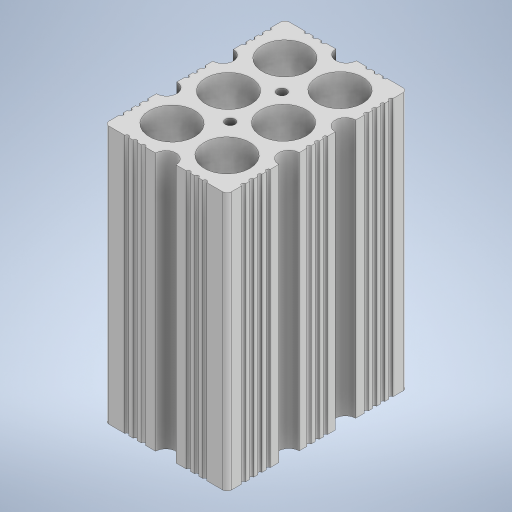
# Autodesk Inventor part: Tijolo 9x19cm
Saved by Autodesk Inventor 2024.4 (Build 284460000, 460)
## iProperties
Created: 2026-08-26
Part Number: Tijolo 9x19cm
Material: Generic
Document SubType Name: Modeling
Designer: MaryPinkAssus
Density: 1 g/cm^3
Appearance: Default
Author: MaryPinkAssus
Autodesk Inventor part; units mm, degrees
ref_plane "YZ Plane" through (0, 0, 0) normal (1, 0, 0) x (0, 1, 0)
ref_plane "XZ Plane" through (0, 0, 0) normal (0, 1, 0) x (-1, 0, 0)
ref_plane "XY Plane" through (0, 0, 0) normal (0, 0, 1) x (1, 0, 0)
sketch "Sketch1" plane through (0, 0, 0) normal (0, 0, 1) x (1, 0, 0)
  line L0 (0, 0) -> (89.5, 0)
  line L1 (89.5, 0) -> (89.5, 188.8)
  line L2 (89.5, 188.8) -> (0, 188.8)
  line L3 (0, 188.8) -> (0, 0)
  dimension "d0" = 89.5
  dimension "d1" = 188.8
  constraints: 8 end point, 2 parallel, 1 horizontal, 1 perpendicular
  measures "d0" distance of L2.end L1.end
  measures "d1" distance of L1.end L0.end
extrude "Corpo" add sketch "Sketch1" along normal blind 131.8
sketch "Furações" plane through (0, 0, 0) normal (0, -1, 0) x (1, 0, 0)
  line L0 (89.5, 131.8) -> (0, 131.8) projected
  line L1 (89.5, 0) -> (0, 0) projected
  line L2 (44.75, 131.8) -> (44.75, 84.8) construction
  line L3 (44.75, 0) -> (44.75, 47) construction
  circle A0 centre (44.75, 84.8) radius 3.5
  circle A1 centre (44.75, 47) radius 3.5
  line L4 (89.5, 123.8) -> (0, 123.8) construction
  line L5 (8, 0) -> (8, 131.8) construction
  line L6 (41.25, 131.8) -> (41.25, 84.8) construction
  circle A2 centre (24.625, 107.175) radius 16.625
  line L7 (0, 0) -> (0, 131.8) construction
  line L8 (0, 65.9) -> (89.5, 65.9) construction
  line L9 (89.5, 0) -> (89.5, 131.8) projected
  line L10 (24.625, 131.8) -> (156.425, 131.8) construction
  circle A3 centre (24.625, 65.9) radius 16.625
  line L11 (0, 8) -> (89.5, 8) construction
  line L12 (41.25, 0) -> (41.25, 47) construction
  circle A4 centre (24.625, 24.625) radius 16.625
  circle A5 centre (64.875, 107.175) radius 16.625
  circle A6 centre (64.875, 65.9) radius 16.625
  circle A7 centre (64.875, 24.625) radius 16.625
  circle A8 centre (44.75, 131.8) radius 7.5
  circle A9 centre (44.75, 0) radius 7.5
  line L13 (24.625, 131.8) -> (24.625, 123.8) construction
  line L14 (24.625, 90.55) -> (24.625, 82.525) construction
  line L15 (24.625, 49.275) -> (24.625, 41.25) construction
  line L16 (24.625, 8) -> (24.625, 0) construction
  line L17 (24.625, 86.5375) -> (0, 86.5375) construction
  line L18 (24.625, 45.2625) -> (0, 45.2625) construction
  circle A10 centre (0, 86.5375) radius 7.5
  circle A11 centre (0, 45.2625) radius 7.5
  circle A12 centre (89.5, 86.5375) radius 7.5
  circle A13 centre (89.5, 45.2625) radius 7.5
  line L19 (0, 123.8) -> (0, 119.8) construction
  circle A14 centre (0, 119.8) radius 1.5
  line L20 (0, 119.8) -> (0, 113.8) construction
  circle A15 centre (0, 113.8) radius 1.5
  line L21 (0, 113.8) -> (0, 107.8) construction
  circle A16 centre (0, 107.8) radius 1.5
  line L22 (0, 107.8) -> (0, 101.8) construction
  circle A17 centre (0, 101.8) radius 1.5
  circle A18 centre (0, 65.9) radius 1.5
  line L23 (0, 65.9) -> (0, 71.9) construction
  line L24 (0, 65.9) -> (0, 59.9) construction
  circle A19 centre (0, 71.9) radius 1.5
  circle A20 centre (0, 59.9) radius 1.5
  line L25 (0, 8) -> (0, 12) construction
  circle A21 centre (0, 12) radius 1.5
  line L26 (0, 12) -> (0, 18) construction
  circle A22 centre (0, 18) radius 1.5
  line L27 (0, 18) -> (0, 24) construction
  circle A23 centre (0, 24) radius 1.5
  line L28 (0, 24) -> (0, 30) construction
  circle A24 centre (0, 30) radius 1.5
  line L29 (37.25, 0) -> (28.25, 0) construction
  circle A25 centre (28.25, 0) radius 1.5
  line L30 (28.25, 0) -> (22.25, 0) construction
  circle A26 centre (22.25, 0) radius 1.5
  line L31 (22.25, 0) -> (16.25, 0) construction
  circle A27 centre (16.25, 0) radius 1.5
  circle A28 centre (28.25, 131.8) radius 1.5
  line L32 (28.25, 131.8) -> (22.25, 131.8) construction
  circle A29 centre (22.25, 131.8) radius 1.5
  line L33 (22.25, 131.8) -> (16.25, 131.8) construction
  circle A30 centre (16.25, 131.8) radius 1.5
  circle A31 centre (89.5, 119.8) radius 1.5
  circle A32 centre (89.5, 113.8) radius 1.5
  circle A33 centre (89.5, 107.8) radius 1.5
  circle A34 centre (89.5, 101.8) radius 1.5
  circle A35 centre (89.5, 65.9) radius 1.5
  circle A36 centre (89.5, 71.9) radius 1.5
  circle A37 centre (89.5, 59.9) radius 1.5
  circle A38 centre (89.5, 12) radius 1.5
  circle A39 centre (89.5, 18) radius 1.5
  circle A40 centre (89.5, 24) radius 1.5
  circle A41 centre (89.5, 30) radius 1.5
  circle A42 centre (61.25, 0) radius 1.5
  circle A43 centre (67.25, 0) radius 1.5
  circle A44 centre (73.25, 0) radius 1.5
  circle A45 centre (73.25, 131.8) radius 1.5
  circle A46 centre (67.25, 131.8) radius 1.5
  circle A47 centre (61.25, 131.8) radius 1.5
  dimension "d4" = 47
  dimension "d5" = 47
  dimension "d6" = 7
  dimension "d7" = 7
  dimension "d8" = 8
  dimension "d9" = 8
  dimension "d10" = 3.5
  dimension "d12" = 33.25
  dimension "d13" = 3.5
  dimension "d14" = 15
  dimension "d15" = 15
  dimension "d16" = 15
  dimension "d17" = 4
  dimension "d18" = 3
  dimension "d19" = 6
  dimension "d20" = 3
  dimension "d21" = 6
  dimension "d22" = 3
  dimension "d23" = 6
  dimension "d24" = 3
  dimension "d25" = 3
  dimension "d26" = 6
  dimension "d27" = 6
  dimension "d28" = 3
  dimension "d29" = 3
  dimension "d30" = 4
  dimension "d31" = 3
  dimension "d32" = 6
  dimension "d33" = 3
  dimension "d34" = 6
  dimension "d35" = 3
  dimension "d36" = 6
  dimension "d37" = 3
  dimension "d38" = 9
  dimension "d39" = 3
  dimension "d40" = 6
  dimension "d41" = 3
  dimension "d42" = 6
  dimension "d43" = 3
  constraints: 60 end point, 47 centre point, 29 symmetric about line, 22 coincident, 6 point on circle, 6 tangent, 4 midpoint, 3 horizontal, 3 parallel, 3 point on line, 2 perpendicular, 1 horizontal alignment, 51 other
  measures "d4" distance of L2.start L2.end
  measures "d5" distance of L3.start L3.end
  measures "d6" diameter of A0
  measures "d7" diameter of A1
  measures "d8" distance between parallel lines of L0 L4
  measures "d9" distance of point (0, 0) L5.start
  measures "d10" distance between parallel lines of L2 L6
  measures "d12" diameter of A3
  measures "d13" distance between parallel lines of L3 L12
  measures "d14" diameter of A8
  measures "d15" diameter of A10
  measures "d16" diameter of A11
  measures "d17" distance of L4.end L19.end
  measures "d18" diameter of A14
  measures "d19" distance of L20.start L20.end
  measures "d20" diameter of A15
  measures "d21" distance of L21.start L21.end
  measures "d22" diameter of A16
  measures "d23" distance of L22.start L22.end
  measures "d24" diameter of A17
  measures "d25" diameter of A18
  measures "d26" distance of L23.start L23.end
  measures "d27" distance of L23.start L24.end
  measures "d28" diameter of A19
  measures "d29" diameter of A20
  measures "d30" distance of L11.start L25.end
  measures "d31" diameter of A21
  measures "d32" distance of L26.start L26.end
  measures "d33" diameter of A22
  measures "d34" distance of L27.start L27.end
  measures "d35" diameter of A23
  measures "d36" distance of L28.start L28.end
  measures "d37" diameter of A24
  measures "d38" distance of L29.start L29.end
  measures "d39" diameter of A25
  measures "d40" distance of L30.start L30.end
  measures "d41" diameter of A26
  measures "d42" distance of L31.start L31.end
  measures "d43" diameter of A27
extrude "furação" cut sketch "Furações" against normal up to surface (188.8 mm away)
fillet "Fillet1" radius 3 4 edges at (0, 94.4, 131.8) (89.5, 94.4, 131.8) (89.5, 94.4, 0) (0, 94.4, 0)
body "Solid1"
